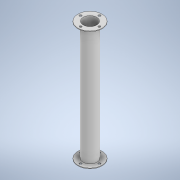
# Autodesk Inventor part: fractionating_column
Saved by Autodesk Inventor 2020 (Build 240168000, 168)
## iProperties
Created: 2022-08-31
Part Number: fractionating_column
Material: Generic
Document SubType Name: Modeling
Designer: Intuito_PC
Density: 1 g/cm^3
Appearance: Default
Author: Intuito_PC
Autodesk Inventor part; units mm, degrees
ref_plane "YZ Plane" through (0, 0, 0) normal (1, 0, 0) x (0, 1, 0)
ref_plane "XZ Plane" through (0, 0, 0) normal (0, 1, 0) x (-1, 0, 0)
sketch "Sketch1" plane through (0, 0, 0) normal (0, 1, 0) x (-1, 0, 0)
  circle A0 centre (0, 0) radius 25
  dimension "d0" = 50
  constraints: 1 centre point, 1 coincident
  measures "d0" diameter of A0
extrude "Extrusion1" add sketch "Sketch1" along normal blind 420
sketch "Sketch2" plane through (0, 420, 0) normal (0, 1, 0) x (1, 0, 0)
  circle A0 centre (0, 0) radius 25 projected
  circle A1 centre (0, 0) radius 24
  dimension "d3" = 48
  constraints: 1 centre point, 1 coincident
  measures "d3" diameter of A1
extrude "Extrusion2" cut sketch "Sketch2" against normal through all contours A1
sketch "Sketch3" plane through (0, 420, 0) normal (0, 1, 0) x (1, 0, 0)
  circle A0 centre (0, 0) radius 43
  dimension "d6" = 86
  constraints: 1 centre point, 1 coincident
  measures "d6" diameter of A0
extrude "Extrusion3" add sketch "Sketch3" along normal blind 2
move faces "Move1" translate (0, 49.2252, 0) faces at (-2.8368, 420, -7.4801)
sketch "Sketch4" plane through (0, 420, 0) normal (0, -1, 0) x (1, 0, 0)
  circle A0 centre (-33.627, 0) radius 4
  point P0 (0, 0)
  dimension "d12" = 8
  constraints: 1 centre point
  measures "d12" diameter of A0
extrude "Extrusion4" cut sketch "Sketch4" against normal blind 2
pattern_circular "Circular Pattern1" count 4 over 360 about axis through (0, 0, 0) along (0, 1, 0) of "Extrusion4"
ref_plane "Work Plane1" through (0, 210, 0) normal (0, -1, 0) x (1, 0, 0)
mirror "Mirror1" about plane through (0, 210, 0) normal (0, -1, 0) of "Extrusion4", "Circular Pattern1", "Extrusion3"
move faces "Move2" translate (0, -46.0502, 0) faces at (-2.8368, 0, -7.4801)
body "Solid1"
